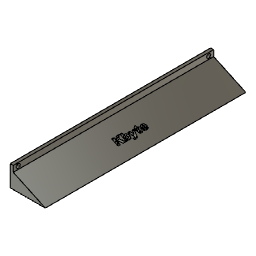
levanta-robo (Autodesk Fusion 360 design; units mm, degrees)
Autodesk Fusion 360 part; units mm, degrees
sketch "Sketch1" plane through (0, 0, 0) normal (0, 1, 0) x (1, 0, 0)
  line L0 (0, 0) -> (35, 0)
  line L1 (0, -20.9218) -> (0, 0)
  line L2 (0, -20.9218) -> (3, -20.9218)
  line L3 (3, -20.9218) -> (3, -14.9218)
  line L4 (3, -14.9218) -> (35, 0)
  dimension "d1" = 35
  dimension "d7" = 3
  dimension "d8" = 25
  dimension "d10" = 6
  constraint coincident L0.start L1.end
  constraint horizontal L0
  constraint perpendicular L0 L1
  constraint perpendicular L1 L2
  constraint perpendicular L2 L3
  measures "d1" distance of L0.start L0.end
  measures "d7" distance of L1.start L2.end
  measures "d8" angle of L0 L4
  measures "d10" distance of L2.end L3.end
extrude "Extrude1" add sketch "Sketch1" along normal blind 200
sketch "Sketch2" plane through (3, 0, 0) normal (1, 0, 0) x (0, 1, 0)
  line L0 (0, 20.9218) -> (0, 14.9218)
  line L1 (0, 14.9218) -> (200, 14.9218)
  line L2 (200, 14.9218) -> (200, 20.9218)
  line L3 (200, 20.9218) -> (0, 20.9218)
  line L4 (10, 20.9218) -> (10, 14.9218)
  line L5 (190, 20.9218) -> (190, 14.9218)
  line L6 (10, 17.9218) -> (0, 17.9218) construction
  line L7 (5, 20.9218) -> (5, 14.9218) construction
  circle A0 centre (5, 17.9218) radius 2
  line L8 (190, 17.9218) -> (200, 17.9218) construction
  line L9 (195, 20.9218) -> (195, 14.9218) construction
  circle A1 centre (195, 17.9218) radius 2
  dimension "d11" = 10
  dimension "d12" = 5
  dimension "d13" = 4
  dimension "d14" = 10
  dimension "d15" = 5
  dimension "d16" = 4
  constraint coincident L3 L4.start
  constraint coincident L1 L4.end
  constraint perpendicular L1 L4
  constraint coincident L3 L5.start
  constraint coincident L1 L5.end
  constraint perpendicular L1 L5
  constraint midpoint L4 L6.start
  constraint midpoint L0 L6.end
  constraint coincident L3 L7.start
  constraint coincident L1 L7.end
  constraint perpendicular L1 L7
  constraint midpoint L6 A0.centre
  constraint midpoint L5 L8.start
  constraint midpoint L2 L8.end
  constraint coincident L3 L9.start
  constraint coincident L1 L9.end
  constraint perpendicular L1 L9
  constraint midpoint L8 A1.centre
  measures "d11" distance of L0 L4
  measures "d12" distance of L4 L7
  measures "d13" diameter of A0
  measures "d14" distance of L2 L5
  measures "d15" distance of L2 L9
  measures "d16" diameter of A1
extrude "Extrude2" cut sketch "Sketch2" against normal blind 3 contours A0 | A1
sketch "Sketch3" plane through (6.2512, 0, 13.4058) normal (0.422618, 0, 0.906308) x (0, 1, 0)
  line L0 (0, 3.5873) -> (0, -31.7208)
  line L1 (0, -31.7208) -> (200, -31.7208)
  line L2 (200, -31.7208) -> (200, 3.5873)
  line L3 (200, 3.5873) -> (0, 3.5873)
  line L4 (84.419, -20.8818) -> (115.5811, -20.8818) construction
  line L5 (115.5811, -20.8818) -> (115.5811, -10.8818) construction
  line L6 (115.5811, -10.8818) -> (84.419, -10.8818) construction
  line L7 (84.419, -10.8818) -> (84.419, -20.8818) construction
  dimension "d19" = 84.419
  dimension "d20" = 10.839
  dimension "d21" = 10
  text T0 "Kbyte" font "Arial Black" height 10 align ink ink in box 0 x 0 at (84.419, -20.8818) x (1, 0) y (0, 1) spacing 1 height is em
  constraint perpendicular L4 L5
  constraint parallel L4 L6
  constraint parallel L5 L7
  measures "d19" distance of L0 L7
  measures "d20" distance of L1 L4
  measures "d21" distance of L4.end L5.end
extrude "Extrude3" cut sketch "Sketch3" against normal blind 5 text T0
